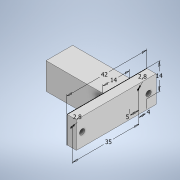
# Autodesk Inventor part: AdaptadorSensorWSMotion
Saved by Autodesk Inventor 2020.3 (Build 243373000, 373)
## iProperties
Created: 2020-09-07
Part Number: AdaptadorSensorWSMotion
Material: Generic
Document SubType Name: Modeling
Designer: mifer
Density: 1 g/cm^3
Appearance: Default
Author: mifer
## iProperties of the stored document _3DPrint.ipt
Created: 2020-09-09
Part Number: _3DPrint
Material: Generic
Document SubType Name: Modeling
Designer: mifer
Density: 1 g/cm^3
Appearance: Default
Author: mifer
Autodesk Inventor part; units mm, degrees
ref_plane "YZ Plane" through (0, 0, 0) normal (1, 0, 0) x (0, 1, 0)
ref_plane "XZ Plane" through (0, 0, 0) normal (0, 1, 0) x (-1, 0, 0)
ref_plane "XY Plane" through (0, 0, 0) normal (0, 0, 1) x (1, 0, 0)
sketch "Sketch1" plane through (0, 0, 0) normal (1, 0, 0) x (0, 1, 0)
  line L0 (0, 0) -> (14, 0)
  line L1 (14, 0) -> (14, -42)
  line L2 (14, -42) -> (0, -42)
  line L3 (0, -42) -> (0, 0)
  line L4 (14, -19) -> (0, -19)
  line L5 (0, -19) -> (0, -33)
  line L6 (0, -33) -> (14, -33)
  line L7 (14, -33) -> (14, -19)
  circle A0 centre (7, -3) radius 1.4
  circle A1 centre (7, -38) radius 1.4
  point P0 (14, -33)
  point P1 (0, -19)
  dimension "d10" = 14
  dimension "d11" = 42
  dimension "d12" = 14
  dimension "d14" = 2.8
  dimension "d15" = 2.8
  dimension "d16" = 35
  dimension "d17" = 4
  dimension "d18" = 5
  constraints: 16 end point, 4 parallel, 2 centre point, 2 horizontal, 2 perpendicular, 2 point on line
  measures "d10" distance of L1.end L2.end
  measures "d11" distance of L0.end L1.end
  measures "d12" distance between parallel lines of L4 L6
  measures "d14" diameter of A0
  measures "d15" diameter of A1
  measures "d16" distance of A1.centre A0.centre
  measures "d17" distance from line of L2 A1.centre
  measures "d18" distance from line of L6 A1.centre
extrude "Extrusion1" add sketch "Sketch1" along normal blind 5 contours L0 L1 L4 L3 | L4 L1 L6 L3 | L6 L1 L2 L3 | A0 | A1
extrude "Extrusion2" add sketch "Sketch1" against normal blind 30 contours L4 L1 L6 L3
sketch "Sketch4" plane through (-30, 0, 0) normal (-1, 0, 0) x (0, 0, 1)
  line L0 (0, 0) -> (-42, 0) projected
  line L1 (-19, 14) -> (-19, 0) projected
  circle A0 centre (-26, 7) radius 1.4
  dimension "d19" = 2.8
  constraints: 1 centre point
  measures "d19" diameter of A0
extrude "Extrusion5" cut sketch "Sketch4" against normal blind 10
extrude "Extrusion6" cut sketch "Sketch1" along normal blind 10 contours A0 | A1
body "Solid1"
